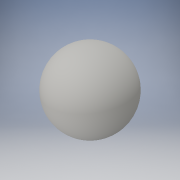
# Autodesk Inventor part: Boulder
Saved by Autodesk Inventor 2016 (Build 200138000, 138)
## iProperties
Created: 2016-01-16
Part Number: Boulder
Material: Generic
Document SubType Name: Modeling
Designer: Mentor1102
Density: 1 g/cm^3
Appearance: Default
Author: Mentor1102
Autodesk Inventor part; units mm, degrees
sketch "Sketch1" plane through (0, 0, 0) normal (0, 0, 1) x (1, 0, 0)
  line L0 (0, 0) -> (254, 0)
  arc A0 (254, 0) -> (0, 0) centre (127, 0) ccw
  dimension "d0" = 254
  dimension "d1" = 127
  constraints: 2 end point, 2 point on circle, 1 centre point, 1 horizontal
  measures "d0" distance of L0.start L0.end
  measures "d1" radius of A0
revolve "Revolution1" add sketch "Sketch1" angle 360 about axis through (0, 0, 0) along (1, 0, 0)
ref_plane "Work Plane1" through (127, 0, 127) normal (0, 0, 1) x (1, 0, 0)
ref_plane "Work Plane2" through (127, 0, -127) normal (0, 0, 1) x (1, 0, 0)
ref_plane "Work Plane4" through (254, 0, 0) normal (1, 0, 0) x (0, 1, 0)
ref_plane "Work Plane5" through (0, 127, 0) normal (0, 1, 0) x (-1, 0, 0)
ref_plane "Work Plane6" through (0, -127, 0) normal (0, 1, 0) x (-1, 0, 0)
ref_plane "Work Plane7" through (127, 0, 0) normal (1, 0, 0) x (0, 1, 0)
body "Solid1"
